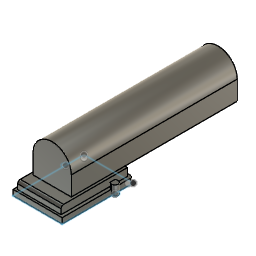
sharpie-adapter (Autodesk Fusion 360 design; units mm, degrees)
Autodesk Fusion 360 part; units mm, degrees
sketch "Sketch1" plane through (0, 0, 0) normal (0, 0, 1) x (1, 0, 0)
  line L0 (-2, 5) -> (15.23, 5)
  line L1 (16.23, 4) -> (16.23, -22.8)
  line L2 (16.23, -22.8) -> (-3, -22.8)
  line L3 (-3, -22.8) -> (-3, 4)
  arc A0 (-2, 5) -> (-3, 4) centre (-2, 4) ccw
  arc A1 (16.23, 4) -> (15.23, 5) centre (15.23, 4) ccw
  arc A2 (-3, -0.9) -> (-3, -3.4) centre (-3, -2.15) ccw
  arc A3 (16.23, -3.4) -> (16.23, -0.9) centre (16.23, -2.15) ccw
  point P0 (-3, 5)
  point P1 (16.23, 5)
  dimension "d1" = 19.23
  dimension "d2" = 27.8
  dimension "d3" = 1
  dimension "d4" = 20.65
  dimension "d5" = 2.5
  dimension "d6" = 2.5
  dimension "d7" = 20.65
  constraint horizontal L0
  constraint vertical L1
  constraint horizontal L2
  constraint vertical L3
  constraint coincident P0 L0
  constraint coincident P0 L3
  constraint tangent L0 A0
  constraint tangent L3 A0
  constraint coincident P1 L0
  constraint coincident P1 L1
  constraint tangent L0 A1
  constraint tangent L1 A1
  constraint equal A0 A1
  constraint coincident L3 A2.centre
  constraint coincident L1 A3.centre
  constraint coincident L3 A2.end
  constraint coincident L3 A2.start
  constraint coincident L1 A3.end
  constraint coincident L1 A3.start
  measures "d1" distance of P0 P1
  measures "d2" distance of P0 L2.end
  measures "d3" radius of A0
  measures "d4" distance of L2.end A2.centre
  measures "d5" diameter of A2
  measures "d6" diameter of A3
  measures "d7" distance of L1.end A3.centre
extrude "Extrude1" add sketch "Sketch1" along normal blind 2.15 contours L0 L1 L2 L3 A0 A1
extrude "Extrude2" add sketch "Sketch1" along normal blind 3.8 contours L3 A2 | L1 A3
sketch "Sketch2" plane through (0, 0, 2.15) normal (0, 0, 1) x (-1, 0, 0)
  line L0 (-16.23, 22.8) -> (-16.23, 3.4)
  arc A0 (-16.23, -4) -> (-15.23, -5) centre (-15.23, -4) ccw
  line L1 (-15.23, -5) -> (2, -5)
  arc A1 (2, -5) -> (3, -4) centre (2, -4) ccw
  line L2 (3, -4) -> (3, 0.9)
  line L3 (3, 22.8) -> (-16.23, 22.8)
  line L4 (2, -4) -> (-15, -4)
  line L5 (-15, -4) -> (-15, 22)
  line L6 (-15, 22) -> (2, 22)
  line L7 (2, 22) -> (2, -4)
  line L8 (-16.23, 3.4) -> (-16.23, 0.9)
  line L9 (-16.23, 0.9) -> (-16.23, -4)
  line L10 (3, 0.9) -> (3, 3.4)
  line L11 (3, 3.4) -> (3, 22.8)
  constraint horizontal L4
  constraint vertical L5
  constraint horizontal L6
  constraint vertical L7
  constraint coincident A1.centre L4.start
extrude "Extrude3" add 1 faces at (-3, -1.7333, 3.25) along direction (1, 0, 0) blind 1
extrude "Extrude4" add 1 faces at (16.23, -1.7333, 2.7) along direction (-1, 0, 0) blind 1
fillet "Fillet1" radius 0.5 2 edges at (-2, -3.4, 2.975) (-2, -0.9, 2.975)
fillet "Fillet2" radius 0.5 2 edges at (15.23, -3.4, 2.975) (15.23, -0.9, 2.975)
extrude "Extrude5" add sketch "Sketch2" along normal blind 3 contours L4 L5 L6 L7
fillet "Fillet3" radius 1 1 edges at (6.5, -22, 5.15)
sketch "Sketch3" plane through (0, 0, 5.15) normal (0, 0, 1) x (-1, 0, 0)
  line L0 (2, 21) -> (-15, 21)
  line L1 (-15, 21) -> (-15, -4)
  line L2 (-15, -4) -> (2, -4)
  line L3 (2, -4) -> (2, 21)
  line L4 (1, 3) -> (-14, 3)
  line L5 (-14, 3) -> (-14, 17)
  line L6 (-14, 17) -> (1, 17)
  line L7 (1, 17) -> (1, 3)
  dimension "d24" = 15
  dimension "d25" = 1
  constraint horizontal L4
  constraint vertical L5
  constraint horizontal L6
  constraint vertical L7
  measures "d24" distance of L4.start L4.end
  measures "d25" distance of L3 L7
extrude "Extrude6" add sketch "Sketch3" along normal blind 15 contours L4 L5 L6 L7
fillet "Fillet4" radius 7.5 2 edges at (-1, -10, 20.15) (14, -10, 20.15)
sketch "Sketch4" plane through (0, -3, 0) normal (0, 1, 0) x (-1, 0, 0)
  arc A0 (1, 12.65) -> (-14, 12.65) centre (-6.5, 12.65) ccw
  line L0 (-14, 12.65) -> (-14, 5.15)
  line L1 (-14, 5.15) -> (1, 5.15)
  line L2 (1, 5.15) -> (1, 12.65)
  circle A1 centre (-6.5, 12.05) radius 6
  dimension "d30" = 12
  dimension "d31" = 7.5
  dimension "d32" = 0.6
  measures "d30" diameter of A1
  measures "d31" distance of L2 A1.centre
  measures "d32" distance of A0.centre A1.centre
extrude "Extrude7" cut sketch "Sketch4" against normal blind 13 contours A1
extrude "Extrude8" add 1 faces at (-0.4111, -3, 9.361) along direction (0, 1, 0) blind 51
